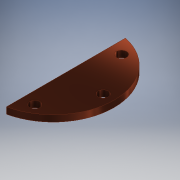
# Autodesk Inventor part: Pulser Plate
Saved by Autodesk Inventor 2017.3 (Build 213256000, 256)
## iProperties
Created: 2017-02-02
Part Number: Pulser Plate
Material: Generic
Document SubType Name: Modeling
Designer: Mac
Density: 1 g/cm^3
Appearance: Copper - Polished
Author: Mac
Autodesk Inventor part; units mm, degrees
ref_plane "YZ Plane" through (0, 0, 0) normal (1, 0, 0) x (0, 1, 0)
ref_plane "XZ Plane" through (0, 0, 0) normal (0, 1, 0) x (-1, 0, 0)
ref_plane "XY Plane" through (0, 0, 0) normal (0, 0, 1) x (1, 0, 0)
sketch "Sketch1" plane through (0, 0, 0) normal (1, 0, 0) x (0, 1, 0)
  circle A0 centre (0, 0) radius 9.5
  dimension "d0" = 19
  constraints: 1 centre point, 1 coincident
  measures "d0" diameter of A0
extrude "Extrusion1" add sketch "Sketch1" along normal blind 1
sketch "Sketch2" plane through (1, 0, 0) normal (1, 0, 0) x (0, 0, -1)
  circle A0 centre (-3.905, 6.7637) radius 0.8
  circle A1 centre (-3.905, -6.7637) radius 0.8
  circle A2 centre (-7.81, 0) radius 0.8
  circle A3 centre (0, 0) radius 9.5 projected
  line L0 (-4.7504, -8.227) -> (14.2614, -8.227) construction
  line L1 (-2, -11) -> (12, -11)
  line L2 (12, -11) -> (12, 10)
  line L3 (12, 10) -> (-2, 10)
  line L4 (-2, 10) -> (-2, -11)
  dimension "d4" = 1.6
  dimension "d8" = 1.6
  dimension "d9" = 1.6
  dimension "d11" = 14
  constraints: 10 end point, 3 centre point, 2 horizontal, 2 parallel, 1 perpendicular, 2 other
  measures "d4" diameter of A0
  measures "d8" diameter of A1
  measures "d9" diameter of A2
  measures "d11" distance of L2.end L3.end
extrude "Extrusion2" cut sketch "Sketch2" against normal blind 1 contours A0 | A1 | A2 | A3 L4 | A3 L4 L3 L2 L1 picked at (1.755, 0.6999)
move or copy body "Move Body1" bodies to move or copy 1 copy no rotation origin (0, 0, 0) rotation axis (0, 1, 0) rotation angle 90 translate (-1, 0, 3)
move or copy body "Move Body2" bodies to move or copy 1 copy no translate (10, 0, 0)
body "Solid1"
